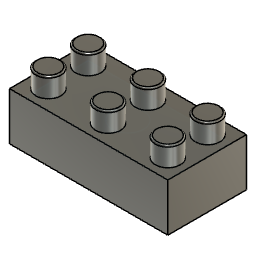
Toy_Block (Autodesk Fusion 360 design; units mm, degrees)
Autodesk Fusion 360 part; units mm, degrees
sketch "Sketch4" plane through (0, 0, 0) normal (0, 0, 1) x (1, 0, 0) in component "2X8 Block1"
  line L0 (0, 0) -> (31.8, 0)
  line L1 (31.8, 0) -> (31.8, 15.8)
  line L2 (31.8, 15.8) -> (0, 15.8)
  line L3 (0, 15.8) -> (0, 0)
  dimension "d23" = 31.8
  dimension "d24" = 15.8
  constraint horizontal L0
  constraint vertical L1
  constraint horizontal L2
  constraint vertical L3
  constraint coincident L0.start L3.end
  measures "d23" distance of L0.start L0.end
  measures "d24" distance of L0.start L2.end
extrude "Extrude4" add sketch "Sketch4" along normal blind 9.6 makes body 1 in component "2X8 Block1"
sketch "Sketch6" plane through (0, 0, 9.6) normal (0, 0, 1) x (-1, 0, 0) in component "2X8 Block1"
  line L0 (0, -15.8) -> (0, 0)
  line L1 (0, 0) -> (-31.8, 0)
  line L2 (-31.8, 0) -> (-31.8, -15.8)
  line L3 (-31.8, -15.8) -> (0, -15.8)
  circle A0 centre (-3.9, -11.9) radius 2.5
  dimension "d28" = 5
  dimension "d31" = 3.9
  dimension "d32" = 3.9
  measures "d28" diameter of A0
  measures "d31" distance of L3 A0.centre
  measures "d32" distance of L0 A0.centre
extrude "Extrude5" add sketch "Sketch6" along normal blind 3.9 separate body contours A0 makes body 2 in component "2X8 Block1"
pattern_linear "R-Pattern3" count 3 spacing 12 along (1, 0, 0) count 2 spacing 8 along (0, -1, 0) of "Extrude5" makes body 3 at (13.4124, 12.1489, 12.2) makes body 4 at (25.4124, 12.1489, 12.2) makes body 5 at (1.4124, 4.1489, 12.2) makes body 6 at (13.4124, 4.1489, 12.2) makes body 7 at (25.4124, 4.1489, 12.2) in component "2X8 Block1"
shell "Shell2" thickness 1.49 removed faces 1 at (21.2, 5.2667, 0) on bodies 1 in component "2X8 Block1"
sketch "Sketch7" plane through (0, 0, 8.11) normal (0, 0, -1) x (1, 0, 0) in component "2X8 Block1"
  line L0 (1.49, -1.49) -> (1.49, -14.31)
  line L1 (1.49, -14.31) -> (30.31, -14.31)
  line L2 (30.31, -14.31) -> (30.31, -1.49)
  line L3 (30.31, -1.49) -> (1.49, -1.49)
  line L4 (1.49, -7.9) -> (34, -7.9) construction
  line L5 (15.9, -14.31) -> (15.9, 1) construction
  circle A0 centre (15.9, -7.9) radius 3.15
  circle A1 centre (15.9, -7.9) radius 2.15
  dimension "d40" = 6.3
  dimension "d41" = -1
  constraint midpoint L0 L4.start
  constraint perpendicular L2 L4
  constraint midpoint L1 L5.start
  constraint perpendicular L3 L5
  constraint coincident L4 A0.centre
  constraint coincident L5 A0.centre
  measures "d40" diameter of A0
extrude "Extrude6" add sketch "Sketch7" along normal blind 8.1 contours A0 bodies 1 in component "2X8 Block1"
sketch "Sketch8" plane through (0, 0, 8.11) normal (0, 0, -1) x (1, 0, 0) in component "2X8 Block1"
  line L0 (1.49, -1.49) -> (1.49, -14.31)
  line L1 (1.49, -14.31) -> (30.31, -14.31)
  line L2 (30.31, -14.31) -> (30.31, -1.49)
  line L3 (30.31, -1.49) -> (1.49, -1.49)
  circle A0 centre (15.9, -7.9) radius 3.15
pattern_linear "R-Pattern4" count 2 spacing 9 along (1, 0, 0) of "Extrude6" in component "2X8 Block1"
pattern_linear "R-Pattern5" count 2 spacing 9 along (-1, 0, 0) of "Extrude6" in component "2X8 Block1"
fillet "Fillet1" radius 0.3 6 edges at (6.2308, 12.804, 13.5) (18.2308, 12.804, 13.5) (30.2308, 12.804, 13.5) (6.2308, 4.804, 13.5) (18.2308, 4.804, 13.5) (30.2308, 4.804, 13.5) on bodies 2 3 4 5 6 7 in component "2X8 Block1"
component "2X8 Block1" placed x (1, 0, 0) y (0, 1, 0) z (0, 0, 1) at (0, 0, 0)
